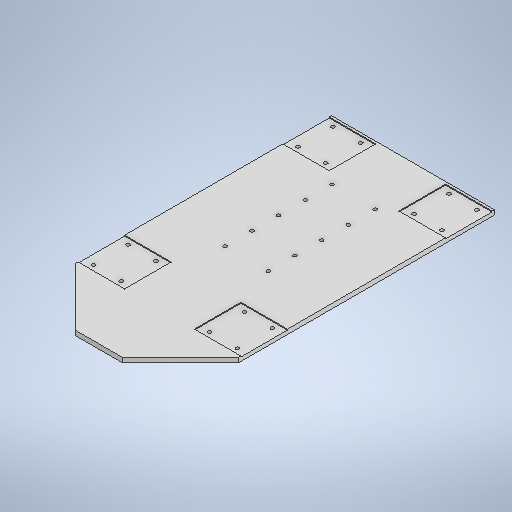
# Autodesk Inventor part: low_base
Saved by Autodesk Inventor 2025 (Build 290162010, 162A)
## iProperties
Created: 2024-10-24
Part Number: low_base
Material: Generic
Document SubType Name: Modeling
Designer: fist5
Density: 1 g/cm^3
Appearance: Default
Author: fist5
Autodesk Inventor part; units mm, degrees
ref_plane "YZ Plane" through (0, 0, 0) normal (1, 0, 0) x (0, 1, 0)
ref_plane "XZ Plane" through (0, 0, 0) normal (0, 1, 0) x (-1, 0, 0)
ref_plane "XY Plane" through (0, 0, 0) normal (0, 0, 1) x (1, 0, 0)
sketch "Sketch1" plane through (0, 0, 0) normal (0, 1, 0) x (-1, 0, 0)
  line L0 (-70, 135) -> (-70, -135)
  line L1 (-70, -135) -> (70, -135)
  line L2 (70, -135) -> (70, 135)
  line L3 (70, 135) -> (-70, 135)
  line L4 (-70, 135) -> (70, -135) construction
  line L5 (-70, -135) -> (70, 135) construction
  line L6 (70, 85) -> (20, 135)
  line L7 (-20, 135) -> (-70, 85)
  point P0 (0, 0)
  dimension "d0" = 140
  dimension "d1" = 270
  dimension "d2" = 40
  dimension "d3" = 50
  dimension "d4" = 220
  constraints: 16 end point, 4 point on line, 2 midpoint, 2 parallel, 1 horizontal alignment, 1 perpendicular, 1 vertical
  measures "d0" distance between parallel lines of L0 L2
  measures "d1" distance between parallel lines of L3 L1
  measures "d2" distance of L7.start L6.end
  measures "d3" distance of L6.end L2.end
  measures "d4" distance of L1.end L6.start
extrude "Extrusion1" add sketch "Sketch1" along normal blind 4.05 and the other way blind 4.05 contours L7 L3 L6 L2 L1 L0
sketch "Sketch2" plane through (0, 0, 0) normal (0, 1, 0) x (-1, 0, 0)
  line L0 (70, -135) -> (70, 85) projected
  line L1 (70, 85) -> (20, 135) projected
  line L2 (20, 135) -> (-20, 135) projected
  line L3 (-20, 135) -> (-70, 85) projected
  line L4 (-70, 85) -> (-70, -135) projected
  line L5 (-70, -135) -> (70, -135) projected
  line L6 (70, 83) -> (30, 83)
  line L7 (30, 83) -> (30, 43)
  line L8 (30, 43) -> (70, 43)
  line L9 (70, 43) -> (70, 83)
  line L10 (70, 85) -> (70, -135) projected
  line L11 (70, -133) -> (30, -133)
  line L12 (30, -133) -> (30, -93)
  line L13 (30, -93) -> (70, -93)
  line L14 (70, -93) -> (70, -133)
  line L15 (-30, 43) -> (-30, 83)
  line L16 (-70, 43) -> (-30, 43)
  line L17 (-30, 83) -> (-70, 83)
  line L18 (-70, 83) -> (-70, 43)
  line L19 (-30, -93) -> (-30, -133)
  line L20 (-70, -93) -> (-30, -93)
  line L21 (-30, -133) -> (-70, -133)
  line L22 (-70, -133) -> (-70, -93)
  point P0 (0, 0)
  point P1 (50, 83)
  point P2 (50, -133)
  point P3 (-50, 83)
  point P4 (-50, -133)
  dimension "d11" = 40
  dimension "d12" = 40
  dimension "d13" = 2
  dimension "d14" = 2
  dimension "d15" = 40
  dimension "d16" = 40
  dimension "d19" = 100
  constraints: 32 end point, 4 parallel, 3 horizontal, 2 midpoint, 2 perpendicular, 2 point on line, 18 other
  measures "d11" distance from line of L8 point (50, 83)
  measures "d12" distance between parallel lines of L7 L0
  measures "d13" distance of L6.start L0.end
  measures "d14" distance between parallel lines of L5 L11
  measures "d15" distance between parallel lines of L12 L0
  measures "d16" distance from line of point (50, -133) L13
  measures "d19" distance of L8.end L15.start
extrude "Extrusion2" cut sketch "Sketch2" along normal blind 0.75 and the other way blind 0.75 contours L11 L12 L13 L0 | L4 L20 L19 L21 | L8 L7 L6 L0 | L4 L17 L15 L16
sketch "Sketch3" plane through (0, 0, 0) normal (0, 1, 0) x (-1, 0, 0)
  line L0 (70, -135) -> (70, 85) projected
  line L1 (70, 85) -> (20, 135) projected
  line L2 (20, 135) -> (-20, 135) projected
  line L3 (-20, 135) -> (-70, 85) projected
  line L4 (-70, 85) -> (-70, -135) projected
  line L5 (-70, -135) -> (70, -135) projected
  point P0 (0, 0)
extrude "Extrusion3" cut sketch "Sketch3" along normal up to surface (4.05 mm away)
sketch "Sketch5" plane through (0, -4.05, 0) normal (0, -1, 0) x (1, 0, 0)
  line L0 (62, 78) -> (38, 78)
  line L1 (38, 78) -> (38, 48)
  line L2 (38, 48) -> (62, 48)
  line L3 (62, 48) -> (62, 78)
  line L4 (30, -93) -> (70, -93) projected
  line L5 (30, -133) -> (30, -93) projected
  line L6 (70, -133) -> (30, -133) projected
  line L7 (70, -135) -> (70, -133) projected
  line L8 (-70, -135) -> (70, -135) projected
  line L9 (-70, -133) -> (-70, -135) projected
  line L10 (-30, -133) -> (-70, -133) projected
  line L11 (-30, -93) -> (-30, -133) projected
  line L12 (-70, -93) -> (-30, -93) projected
  line L13 (-70, 43) -> (-70, -93) projected
  line L14 (-30, 43) -> (-70, 43) projected
  line L15 (-30, 83) -> (-30, 43) projected
  line L16 (-70, 83) -> (-30, 83) projected
  line L17 (-70, 85) -> (-70, 83) projected
  line L18 (-20, 135) -> (-70, 85) projected
  line L19 (20, 135) -> (-20, 135) projected
  line L20 (70, 85) -> (20, 135) projected
  line L21 (70, 83) -> (70, 85) projected
  line L22 (30, 83) -> (70, 83) projected
  line L23 (30, 43) -> (30, 83) projected
  line L24 (70, 43) -> (30, 43) projected
  line L25 (70, -93) -> (70, 43) projected
  circle A0 centre (62, 78) radius 1.5
  point P0 (0, 0)
  dimension "d31" = 24
  dimension "d32" = 30
  dimension "d33" = 8
  dimension "d34" = 5
  dimension "d35" = 3
  constraints: 8 end point, 2 parallel, 1 centre point, 1 coincident, 1 horizontal, 1 perpendicular
  measures "d31" distance between parallel lines of L1 L3
  measures "d32" distance between parallel lines of L2 L0
  measures "d33" distance between parallel lines of L23 L1
  measures "d34" distance between parallel lines of L24 L2
  measures "d35" diameter of A0
extrude "Extrusion4" cut sketch "Sketch5" against normal up to surface (3.3 mm away) contours L3 A0 L0 | L0 A0 L3
pattern_linear "Rectangular Pattern1" count 2 spacing 30 along (0, 0, -1) count 2 spacing 24 along (-1, 0, 0) of "Extrusion4"
pattern_linear "Rectangular Pattern2" count 2 spacing 176 along (0, 0, -1) count 2 spacing 100 along (-1, 0, 0) of "Extrusion4", "Rectangular Pattern1"
sketch "Sketch6" plane through (0, -4.05, 0) normal (0, -1, 0) x (1, 0, 0)
  line L0 (18.5, -84) -> (-18.5, -84)
  line L1 (-18.5, -84) -> (-18.5, 8)
  line L2 (-18.5, 8) -> (18.5, 8)
  line L3 (18.5, 8) -> (18.5, -84)
  line L4 (70, -93) -> (70, 43) projected
  line L5 (70, 13) -> (-70, 13)
  line L6 (-70, 85) -> (-70, -135) projected
  line L7 (-70, -135) -> (70, -135) projected
  circle A0 centre (18.5, 8) radius 1.5
  point P0 (0, 0)
  point P1 (0, 8)
  dimension "d50" = 148
  dimension "d51" = 5
  dimension "d52" = 92
  dimension "d53" = 37
  dimension "d54" = 3
  constraints: 10 end point, 2 horizontal, 2 parallel, 2 point on line, 1 centre point, 1 coincident, 1 midpoint, 1 perpendicular, 1 vertical alignment
  measures "d50" distance between parallel lines of L7 L5
  measures "d51" distance between parallel lines of L5 L2
  measures "d52" distance from line of L0 point (0, 8)
  measures "d53" distance between parallel lines of L1 L3
  measures "d54" diameter of A0
extrude "Extrusion5" cut sketch "Sketch6" against normal up to next contours A0 L2 L3 | L3 L2 A0
pattern_linear "Rectangular Pattern3" count 5 spacing 23 along (0, 0, -1) count 2 spacing 37 along (-1, 0, 0) of "Extrusion5"
body "Solid1"
